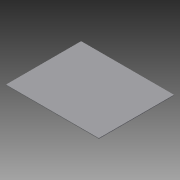
# Autodesk Inventor part: liftingMechanismPlate
Saved by Autodesk Inventor 2015 (Build 190159000, 159)
## iProperties
Created: 2015-01-30
Part Number: liftingMechanismPlate
Material: Generic
Document SubType Name: Modeling
Designer: Kingbob26
Density: 1 g/cm^3
Appearance: Default
Author: Kingbob26
Autodesk Inventor part; units mm, degrees
ref_plane "YZ Plane" through (0, 0, 0) normal (1, 0, 0) x (0, 1, 0)
ref_plane "XZ Plane" through (0, 0, 0) normal (0, 1, 0) x (-1, 0, 0)
ref_plane "XY Plane" through (0, 0, 0) normal (0, 0, 1) x (1, 0, 0)
sketch "Sketch1" plane through (0, 0, 0) normal (0, 1, 0) x (-1, 0, 0)
  line L0 (494.3094, 400.05) -> (0, 400.05)
  line L1 (0, 400.05) -> (0, 0)
  line L2 (0, 0) -> (494.3094, 0)
  line L3 (494.3094, 0) -> (494.3094, 400.05)
  constraints: 8 end point, 2 parallel, 1 horizontal, 1 perpendicular
extrude "Extrusion1" add sketch "Sketch1" along normal blind 3.175
fillet "Fillet1" radius 3.175 1 edges at (0, 1.5875, 400.05)
fillet "Fillet2" radius 3.175 1 edges at (0, 1.5875, 0)
fillet "Fillet3" radius 3.175 1 edges at (-494.3094, 1.5875, 0)
fillet "Fillet4" radius 3.175 1 edges at (-494.3094, 1.5875, 400.05)
body "Solid1"
